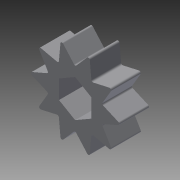
# Autodesk Inventor part: 000113
Saved by Autodesk Inventor 2015 (Build 190159000, 159)
## iProperties
Created: 2015-05-13
Part Number: 000113
Material: Generic
Document SubType Name: Modeling
Designer: Wesley
Density: 1 g/cm^3
Appearance: Default
Author: Wesley
Autodesk Inventor part; units mm, degrees
ref_plane "YZ Plane" through (0, 0, 0) normal (1, 0, 0) x (0, 1, 0)
ref_plane "XZ Plane" through (0, 0, 0) normal (0, 1, 0) x (-1, 0, 0)
ref_plane "XY Plane" through (0, 0, 0) normal (0, 0, 1) x (1, 0, 0)
sketch "Sketch1" plane through (0, 0, 0) normal (0, 0, 1) x (1, 0, 0)
  circle A0 centre (0, 0) radius 2.3812 construction
  circle A1 centre (0, 0) radius 3.9687 construction
  circle A2 centre (0, 0) radius 2.3812
  circle A3 centre (0, 0) radius 2.3812
  circle A4 centre (0, 0) radius 2.3812
  circle A5 centre (0, 0) radius 2.3812
  circle A6 centre (0, 0) radius 2.3812
  circle A7 centre (0, 0) radius 2.3812
  circle A8 centre (0, 0) radius 2.3812
  circle A9 centre (0, 0) radius 2.3812
  circle A10 centre (0, 0) radius 2.3812
  line L0 (-1.3997, 1.9265) -> (-1.2264, 3.7745)
  line L1 (-1.2264, 3.7745) -> (0, 2.3812)
  line L2 (1.3997, 1.9265) -> (3.2108, 2.3328)
  line L3 (3.2108, 2.3328) -> (2.2647, 0.7358)
  line L4 (3.9687, 0) -> (2.2647, 0.7358)
  line L5 (3.9687, 0) -> (2.2647, -0.7358)
  line L6 (3.2108, -2.3328) -> (2.2647, -0.7358)
  line L7 (1.3997, -1.9265) -> (3.2108, -2.3328)
  line L8 (1.3997, -1.9265) -> (1.2264, -3.7745)
  line L9 (1.2264, -3.7745) -> (0, -2.3812)
  line L10 (-1.2264, -3.7745) -> (0, -2.3812)
  line L11 (-1.3997, -1.9265) -> (-1.2264, -3.7745)
  line L12 (-1.3997, -1.9265) -> (-3.2108, -2.3328)
  line L13 (-3.2108, -2.3328) -> (-2.2647, -0.7358)
  line L14 (-2.2647, -0.7358) -> (-3.9687, 0)
  line L15 (-3.9687, 0) -> (-2.2647, 0.7358)
  line L16 (-3.2108, 2.3328) -> (-2.2647, 0.7358)
  line L17 (-3.2108, 2.3328) -> (-1.3997, 1.9265)
  line L18 (0, 2.3812) -> (1.2264, 3.7745)
  line L19 (1.2264, 3.7745) -> (1.3997, 1.9265)
  dimension "d0" = 4.7625
  dimension "d1" = 7.9375
  dimension "d4" = 360
  dimension "d6" = 82.712
  constraints: 40 end point, 13 coincident, 2 vertical alignment, 1 horizontal alignment, 78 other
  measures "d6" angle of L18 L1
extrude "Extrusion1" add sketch "Sketch1" along normal blind 2.54
sketch "Sketch2" plane through (0, 0, 2.54) normal (0, 0, 1) x (1, 0, 0)
  line L0 (0, 1.5926) -> (1.3792, 0.7963)
  line L1 (1.3792, 0.7963) -> (1.3792, -0.7963)
  line L2 (1.3792, -0.7963) -> (0, -1.5926)
  line L3 (0, -1.5926) -> (-1.3792, -0.7963)
  line L4 (-1.3792, -0.7963) -> (-1.3792, 0.7963)
  line L5 (-1.3792, 0.7963) -> (0, 1.5926)
  point P0 (0, 0)
  point P1 (0, 0)
  dimension "d9" = 3.1852
  dimension "d10" = 1.3792
  constraints: 12 end point, 1 coincident, 13 other
  measures "d9" distance of L2.end L0.start
  measures "d10" horizontal distance of L1.end L2.end
extrude "Extrusion2" cut sketch "Sketch2" against normal through all
fillet "Fillet1" radius 0.127 20 edges at (-3.2108, -2.3328, 1.27) (-3.9687, 0, 1.27) (-3.2108, 2.3328, 1.27) (-1.2264, 3.7745, 1.27) (1.2264, 3.7745, 1.27) (3.2108, 2.3328, 1.27) (3.9687, 0, 1.27) (3.2108, -2.3328, 1.27) (1.2264, -3.7745, 1.27) (-1.2264, -3.7745, 1.27) (0, -2.3812, 1.27) (1.3997, -1.9265, 1.27) (2.2647, 0.7358, 1.27) (2.2647, -0.7358, 1.27) (1.3997, 1.9265, 1.27) (0, 2.3812, 1.27) (-1.3997, 1.9265, 1.27) (-2.2647, 0.7358, 1.27) (-2.2647, -0.7358, 1.27) (-1.3997, -1.9265, 1.27)
body "Solid1"
